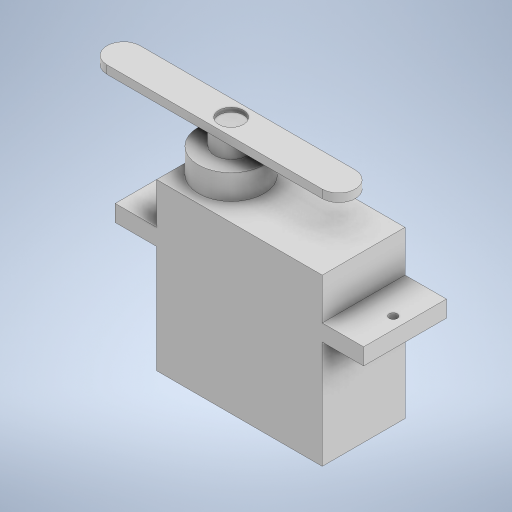
# Autodesk Inventor part: servo
Saved by Autodesk Inventor 2023 (Build 270158000, 158)
## iProperties
Created: 2023-01-20
Part Number: servo
Material: Generic
Document SubType Name: Modeling
Designer: kavya
Density: 1 g/cm^3
Appearance: Default
Author: kavya
Autodesk Inventor part; units mm, degrees
ref_plane "YZ Plane" through (0, 0, 0) normal (1, 0, 0) x (0, 1, 0)
ref_plane "XZ Plane" through (0, 0, 0) normal (0, 1, 0) x (-1, 0, 0)
ref_plane "XY Plane" through (0, 0, 0) normal (0, 0, 1) x (1, 0, 0)
sketch "Sketch1" plane through (0, 0, 0) normal (0, 0, 1) x (1, 0, 0)
  line L0 (0, 0) -> (20, 0)
  line L1 (20, 0) -> (20, 20)
  line L2 (20, 20) -> (0, 20)
  line L3 (0, 20) -> (0, 0)
  dimension "d0" = 20
  dimension "d1" = 20
  constraints: 8 end point, 2 parallel, 1 horizontal, 1 perpendicular
  measures "d0" distance of L2.end L1.end
  measures "d1" distance of L1.end L0.end
extrude "Extrusion1" add sketch "Sketch1" along normal blind 10
sketch "Sketch2" plane through (20, 0, 0) normal (1, 0, 0) x (0, 0, -1)
  line L0 (0, 0) -> (0, 20) projected
  line L1 (0, 15) -> (-10, 15)
  line L2 (-10, 15) -> (-10, 13)
  line L3 (-10, 13) -> (0, 13)
  line L4 (0, 13) -> (0, 15)
  dimension "d4" = 10
  dimension "d5" = 2
  constraints: 8 end point, 2 parallel, 1 horizontal, 1 perpendicular, 1 point on line
  measures "d4" distance of L3.end L2.end
  measures "d5" distance of L2.end L1.end
extrude "Extrusion2" add sketch "Sketch2" along normal blind 5
sketch "Sketch3" plane through (0, 0, 0) normal (-1, 0, 0) x (0, 0, 1)
  line L0 (10, 15) -> (10, 13) projected
  line L1 (0, 15) -> (10, 15)
  line L2 (10, 15) -> (10, 13)
  line L3 (10, 13) -> (0, 13)
  line L4 (0, 13) -> (0, 15)
  point P0 (0, 0)
  dimension "d8" = 2
  constraints: 8 end point, 2 parallel, 1 horizontal, 1 perpendicular
  measures "d8" distance of L1.end L0.end
extrude "Extrusion3" add sketch "Sketch3" along normal blind 5
sketch "Sketch4" plane through (20, 15, 10) normal (0, 1, 0) x (1, 0, 0)
  circle A0 centre (-23.5755, 5) radius 0.5
  line L0 (0, 10) -> (-20, 10) projected
  line L1 (-10, 10) -> (-10, 0.1248)
  line L2 (-10, 0.1248) -> (-10, 10)
  circle A1 centre (3.5755, 5) radius 0.5
  dimension "d11" = 1
  constraints: 4 end point, 2 centre point, 1 collinear, 1 midpoint, 1 symmetric about line, 1 vertical, 1 other
  measures "d11" diameter of A0
extrude "Extrusion4" cut sketch "Sketch4" against normal through all
sketch "Sketch5" plane through (0, 20, 0) normal (0, 1, 0) x (1, 0, 0)
  circle A0 centre (4, -5) radius 3.9548
  point P0 (0, 0)
  constraints: 1 centre point
extrude "Extrusion5" add sketch "Sketch5" along normal blind 3
sketch "Sketch6" plane through (4, 23, 5) normal (0, 1, 0) x (1, 0, 0)
  circle A0 centre (0, 0) radius 2
  point P0 (-4, 5)
  dimension "d16" = 4
  constraints: 1 centre point
  measures "d16" diameter of A0
extrude "Extrusion6" add sketch "Sketch6" along normal blind 2
sketch "Sketch7" plane through (4, 25, 5) normal (0, 1, 0) x (1, 0, 0)
  circle A0 centre (0, 0) radius 2 projected
  line L0 (0, 2) -> (13, 2)
  line L1 (15, 0) -> (15, 0)
  line L2 (13, -2) -> (0, -2)
  line L3 (0, -2) -> (0, 2)
  line L4 (0, 2) -> (-13, 2)
  line L5 (-15, 0) -> (-15, 0)
  line L6 (-13, -2) -> (0, -2)
  line L7 (0, -2) -> (0, 2)
  arc A1 (-13, 2) -> (-15, 0) centre (-13, 0) ccw
  arc A2 (-15, 0) -> (-13, -2) centre (-13, 0) ccw
  arc A3 (13, -2) -> (15, 0) centre (13, 0) ccw
  arc A4 (15, 0) -> (13, 2) centre (13, 0) ccw
  point P0 (-4, 5)
  point P1 (15, -2)
  point P2 (-15, -2)
  point P3 (0, -2)
  point P4 (15, 0)
  dimension "d19" = 15
  dimension "d20" = 15
  dimension "d21" = 2
  constraints: 16 end point, 8 point on circle, 8 tangent, 5 point on line, 4 centre point, 4 parallel, 3 equal radius, 2 horizontal, 2 perpendicular, 1 vertical alignment, 1 other
  measures "d19" distance of point (15, -2) L2.end
  measures "d20" distance of L6.end point (-15, -2)
  measures "d21" radius of A1
extrude "Extrusion7" add sketch "Sketch7" along normal blind 1
sketch "Sketch8" plane through (4, 26, 5) normal (0, 1, 0) x (1, 0, 0)
  circle A0 centre (0, 0) radius 1.5
  point P0 (-4, 5)
  dimension "d24" = 3
  constraints: 1 centre point
  measures "d24" diameter of A0
extrude "Extrusion8" cut sketch "Sketch8" against normal blind 0.5
body "Solid1"
